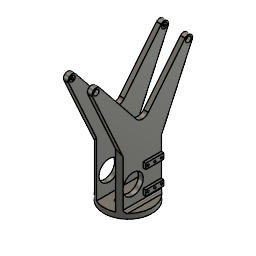
Base plate PiPER v7 V2 (Autodesk Fusion 360 design; units mm, degrees)
part number: 2025-11-21-17-17-18-129
Autodesk Fusion 360 part; units mm, degrees
sketch "Sketch1" plane through (0, 0, 0) normal (0, 1, 0) x (1, 0, 0)
  circle A0 centre (0, 0) radius 28.5
  circle A1 centre (11.6913, -6.75) radius 2
  circle A2 centre (11.6913, 6.75) radius 2
  circle A3 centre (0, 13.5) radius 2
  circle A4 centre (-11.6913, 6.75) radius 2
  circle A5 centre (-11.6913, -6.75) radius 2
  circle A6 centre (0, -13.5) radius 2
  spline S0 degree 5 poles (2.6699, 14.6244) (2.6558, 14.5371) (2.6371, 14.3587) (2.6331, 14.0815) (2.6571, 13.7017) (2.6824, 13.2287) (2.655, 12.7724) (2.5426, 12.3428) (2.3408, 11.943) (2.0817, 11.5691) (1.8161, 11.2121) (1.5972, 10.8601) (1.4651, 10.5006) (1.4272, 10.1227) (1.4558, 9.719) (1.5099, 9.2874) (1.5508, 8.8329) (1.5594, 8.369) (1.5542, 7.9199) (1.5754, 7.5127) (1.6684, 7.1694) (1.868, 6.8996) (2.1791, 6.6899) (2.5766, 6.5084) (3.0214, 6.3189) (3.4712, 6.0933) (3.8935, 5.8234) (4.2785, 5.5351) (4.6335, 5.2747) (4.9749, 5.0918) (5.3217, 5.0256) (5.6878, 5.086) (6.0765, 5.2462) (6.4838, 5.4621) (6.8992, 5.6875) (7.3078, 5.8897) (7.692, 6.069) (8.0346, 6.2519) (8.3242, 6.4724) (8.5585, 6.7591) (8.7505, 7.1166) (8.9281, 7.5201) (9.1243, 7.9319) (9.3686, 8.3127) (9.6795, 8.6342) (10.0543, 8.8943) (10.4711, 9.1133) (10.896, 9.3237) (11.2884, 9.5617) (11.6068, 9.8592) (11.815, 10.2333) (11.8842, 10.6878) (11.7936, 11.2159) (11.5324, 11.8027) (11.1006, 12.4275) (10.5109, 13.0664) (9.7861, 13.6938) (8.957, 14.2835) (8.0599, 14.8102) (7.1342, 15.2509) (6.2204, 15.5861) (5.3571, 15.801) (4.5795, 15.8872) (3.9162, 15.8439) (3.3874, 15.6792) (3.003, 15.4088) (2.8094, 15.1239) (2.7213, 14.8822) (2.6839, 14.7116) (2.6699, 14.6244) knots 0 0 0 0 0 0 0.01538462 0.03076923 0.04615385 0.06153846 0.07692308 0.09230769 0.10769231 0.12307692 0.13846154 0.15384615 0.16923077 0.18461538 0.2 0.21538462 0.23076923 0.24615385 0.26153846 0.27692308 0.29230769 0.30769231 0.32307692 0.33846154 0.35384615 0.36923077 0.38461538 0.4 0.41538462 0.43076923 0.44615385 0.46153846 0.47692308 0.49230769 0.50769231 0.52307692 0.53846154 0.55384615 0.56923077 0.58461538 0.6 0.61538462 0.63076923 0.64615385 0.66153846 0.67692308 0.69230769 0.70769231 0.72307692 0.73846154 0.75384615 0.76923077 0.78461538 0.8 0.81538462 0.83076923 0.84615385 0.86153846 0.87692308 0.89230769 0.90769231 0.92307692 0.93846154 0.95384615 0.96923077 0.98461538 1 1 1 1 1 1
  spline S1 degree 5 poles (-14, -5) (-13.9174, -4.9685) (-13.7535, -4.8955) (-13.5115, -4.7604) (-13.1946, -4.5497) (-12.7976, -4.2913) (-12.3888, -4.0869) (-11.9605, -3.9694) (-11.5134, -3.9443) (-11.06, -3.9818) (-10.618, -4.0333) (-10.2037, -4.0469) (-9.8264, -3.9814) (-9.4801, -3.8253) (-9.1448, -3.5987) (-8.7981, -3.3361) (-8.4249, -3.0734) (-8.0275, -2.834) (-7.6359, -2.614) (-7.2939, -2.392) (-7.0431, -2.1399) (-6.9092, -1.8321) (-6.8831, -1.4578) (-6.9247, -1.0228) (-6.9831, -0.5428) (-7.0126, -0.0405) (-6.99, 0.4602) (-6.9328, 0.9377) (-6.8848, 1.3754) (-6.8971, 1.7624) (-7.0131, 2.096) (-7.2485, 2.3828) (-7.5816, 2.6393) (-7.9722, 2.8841) (-8.3751, 3.1311) (-8.7545, 3.3839) (-9.1019, 3.6269) (-9.4316, 3.8323) (-9.7674, 3.9728) (-10.1328, 4.0323) (-10.5384, 4.0199) (-10.9767, 3.9719) (-11.4313, 3.9359) (-11.8832, 3.9571) (-12.3172, 4.0656) (-12.7299, 4.2601) (-13.1279, 4.5116) (-13.5225, 4.7744) (-13.9249, 4.9951) (-14.3417, 5.1222) (-14.7698, 5.1155) (-15.198, 4.9481) (-15.6101, 4.6056) (-15.9876, 4.086) (-16.3128, 3.3996) (-16.5713, 2.5695) (-16.7522, 1.6281) (-16.8484, 0.6152) (-16.856, -0.4251) (-16.7748, -1.4471) (-16.6081, -2.406) (-16.3626, -3.2611) (-16.0484, -3.9776) (-15.6793, -4.5304) (-15.2723, -4.9061) (-14.8459, -5.1037) (-14.5024, -5.129) (-14.249, -5.0843) (-14.0826, -5.0315) (-14, -5) knots 0 0 0 0 0 0 0.01538462 0.03076923 0.04615385 0.06153846 0.07692308 0.09230769 0.10769231 0.12307692 0.13846154 0.15384615 0.16923077 0.18461538 0.2 0.21538462 0.23076923 0.24615385 0.26153846 0.27692308 0.29230769 0.30769231 0.32307692 0.33846154 0.35384615 0.36923077 0.38461538 0.4 0.41538462 0.43076923 0.44615385 0.46153846 0.47692308 0.49230769 0.50769231 0.52307692 0.53846154 0.55384615 0.56923077 0.58461538 0.6 0.61538462 0.63076923 0.64615385 0.66153846 0.67692308 0.69230769 0.70769231 0.72307692 0.73846154 0.75384615 0.76923077 0.78461538 0.8 0.81538462 0.83076923 0.84615385 0.86153846 0.87692308 0.89230769 0.90769231 0.92307692 0.93846154 0.95384615 0.96923077 0.98461538 1 1 1 1 1 1
  spline S2 degree 5 poles (11.3301, -9.6244) (11.2616, -9.5686) (11.1164, -9.4631) (10.8784, -9.3211) (10.5375, -9.152) (10.1152, -8.9374) (9.7338, -8.6855) (9.4179, -8.3733) (9.1726, -7.9987) (8.9783, -7.5873) (8.8019, -7.1788) (8.6066, -6.8132) (8.3612, -6.5192) (8.0529, -6.2973) (7.689, -6.1203) (7.2882, -5.9514) (6.8741, -5.7595) (6.4681, -5.535) (6.0817, -5.3059) (5.7185, -5.1207) (5.3747, -5.0296) (5.0412, -5.0675) (4.7041, -5.2321) (4.3481, -5.4856) (3.9617, -5.7761) (3.5414, -6.0528) (3.0965, -6.2836) (2.6543, -6.4729) (2.2513, -6.6501) (1.9222, -6.8543) (1.6914, -7.1215) (1.5607, -7.4688) (1.5051, -7.8856) (1.4884, -8.3462) (1.4759, -8.8186) (1.4467, -9.2736) (1.4099, -9.696) (1.397, -10.0842) (1.4432, -10.4452) (1.5743, -10.7914) (1.7879, -11.1365) (2.0486, -11.4921) (2.3071, -11.8678) (2.5147, -12.2697) (2.6377, -12.6998) (2.6756, -13.1545) (2.6568, -13.6249) (2.6265, -14.098) (2.6365, -14.5569) (2.7349, -14.9813) (2.9548, -15.3487) (3.3138, -15.6359) (3.8165, -15.8215) (4.4553, -15.8887) (5.2122, -15.8272) (6.0604, -15.6359) (6.9661, -15.3219) (7.8914, -14.8987) (8.7961, -14.3852) (9.6406, -13.8039) (10.3878, -13.18) (11.0055, -12.5399) (11.4689, -11.9095) (11.7631, -11.3134) (11.8849, -10.7732) (11.8429, -10.305) (11.693, -9.995) (11.5277, -9.7978) (11.3987, -9.6801) (11.3301, -9.6244) knots 0 0 0 0 0 0 0.01538462 0.03076923 0.04615385 0.06153846 0.07692308 0.09230769 0.10769231 0.12307692 0.13846154 0.15384615 0.16923077 0.18461538 0.2 0.21538462 0.23076923 0.24615385 0.26153846 0.27692308 0.29230769 0.30769231 0.32307692 0.33846154 0.35384615 0.36923077 0.38461538 0.4 0.41538462 0.43076923 0.44615385 0.46153846 0.47692308 0.49230769 0.50769231 0.52307692 0.53846154 0.55384615 0.56923077 0.58461538 0.6 0.61538462 0.63076923 0.64615385 0.66153846 0.67692308 0.69230769 0.70769231 0.72307692 0.73846154 0.75384615 0.76923077 0.78461538 0.8 0.81538462 0.83076923 0.84615385 0.86153846 0.87692308 0.89230769 0.90769231 0.92307692 0.93846154 0.95384615 0.96923077 0.98461538 1 1 1 1 1 1
  circle A7 centre (0, 0) radius 13.5 construction
  circle A8 centre (0, -13.5) radius 1.7
  circle A9 centre (0, 13.5) radius 1.7
  line L0 (-7, 0) -> (-16.8414, 0) construction
  circle A10 centre (-11.9207, 0) radius 2.1654
  circle A11 centre (5.9604, -10.3236) radius 2.1654
  circle A12 centre (5.9604, 10.3236) radius 2.1654
  point P0 (2.5359, 12.3923)
  point P1 (1.5359, 10.6603)
  point P2 (1.7679, 7.0622)
  point P3 (5.2321, 5.0622)
  point P4 (8.4641, 6.6603)
  point P5 (9.4641, 8.3923)
  point P6 (11.3301, 9.6244)
  point P7 (11.4641, 11.8564)
  point P8 (4.5359, 15.8564)
  point P9 (3.5, 6.0622)
  point P10 (7.0147, 5.7421)
  point P11 (1.5439, 8.8149)
  point P12 (-12, -4)
  point P13 (-10, -4)
  point P14 (-8.4059, -3.0704)
  point P15 (-7, -2)
  point P16 (-7, 0)
  point P17 (-7, 2)
  point P18 (-8.4801, 3.2039)
  point P19 (-10, 4)
  point P20 (-12, 4)
  point P21 (-14, 5)
  point P22 (-16, 4)
  point P23 (-16, -4)
  point P24 (9.4641, -8.3923)
  point P25 (8.4641, -6.6603)
  point P26 (6.862, -5.7445)
  point P27 (5.2321, -5.0622)
  point P28 (3.5, -6.0622)
  point P29 (1.7679, -7.0622)
  point P30 (1.4654, -8.946)
  point P31 (1.5359, -10.6603)
  point P32 (2.5359, -12.3923)
  point P33 (2.6699, -14.6244)
  point P34 (4.5359, -15.8564)
  point P35 (11.4641, -11.8564)
  dimension "d3" = 57
  dimension "d9" = 4
  dimension "d11" = 360
  dimension "d33" = 27
  dimension "d255" = 3.4
  dimension "d256" = 3.4
  constraint coincident A0.centre A7.centre
  constraint concentric A0 A7
  constraint concentric A6 A8
  constraint concentric A3 A9
  constraint coincident P16 L0.start
  constraint coincident S1 L0.end
  constraint horizontal L0
  constraint midpoint L0 A10.centre
  measures "d3" diameter of A0
  measures "d9" diameter of A1
  measures "d33" diameter of A7
  measures "d255" diameter of A8
  measures "d256" diameter of A9
extrude "Extrude7" add sketch "Sketch1" against normal blind 4 contours S0 | S1 | S2 | A10 | A11 | A12 makes body 1 at (9.8365, -1.0048, 8.738) makes body 2 at (-12.8395, -1.0048, -4.3378) makes body 3 at (2.6491, -1.0048, -12.8883)
scale "Scale1" factor 1 about (-14, -4, 5) bodies 2
scale "Scale2" factor 0.9 about (-11.9207, 0, 0) bodies 2
scale "Scale3" factor 0.9 about (5.9604, 0, 10.3236) bodies 1
scale "Scale4" factor 0.9 about (5.9604, 0, -10.3236) bodies 3
extrude "Extrude35" add sketch "Sketch1" along normal blind 2 separate body contours A3 | A6 makes body 4 at (1.9975, 1.3333, -13.4003) makes body 5 at (1.9975, 1.3333, 13.5997)
extrude "Extrude24" add sketch "Sketch1" along normal blind 6 contours A0 | A1 | A2 | A4 | A5 | S0 | S1 | S2 | A10 | A11 | A12 bodies 1 4 5 2 3
sketch "Sketch13" plane through (0, 6, 0) normal (0, 1, 0) x (-1, 0, 0)
  circle A0 centre (0, -13.5) radius 2
  circle A1 centre (0, 13.5) radius 2
  line L0 (0, 0) -> (9, 0)
  line L1 (14, 0) -> (14, -21.9089)
  line L2 (14, 0) -> (14, 21.9089)
  line L3 (0, 40) -> (0, -40)
  line L4 (-14, 0) -> (-14, 21.9089)
  line L5 (-14, 0) -> (-14, -21.9089)
  line L6 (8.9562, 50) -> (17.0461, 50)
  line L7 (17.0461, 50) -> (17.0461, -50)
  line L8 (17.0461, -50) -> (11.4128, -50)
  line L9 (-8.9562, 50) -> (-17.0461, 50)
  line L10 (-17.0461, 50) -> (-17.0461, -50)
  line L11 (-17.0461, -50) -> (-11.4128, -50)
  circle A2 centre (0, 0) radius 28.5
  line L12 (-11.4128, 50.6271) -> (-11.4128, -50)
  line L13 (11.4128, 50.6271) -> (11.4128, -50)
  line L14 (0, -40) -> (-11.5, -40) construction
  line L15 (-11.5, -40) -> (-17.044, -40)
  dimension "d228" = 5.544
  constraint coincident L0.start A2.centre
  constraint horizontal L0
  constraint perpendicular L0 L1
  constraint parallel L1 L2
  constraint vertical L3
  constraint symmetric L1.start L3 L4.start
  constraint symmetric L1.end L3 L5.end
  constraint symmetric L2.end L3 L4.end
  constraint horizontal L6
  constraint vertical L7
  constraint horizontal L8
  constraint symmetric L3 L6.start L9.start
  constraint symmetric L3 L6.end L9.end
  constraint symmetric L3 L7.end L10.end
  constraint symmetric L3 L8.end L11.end
  constraint perpendicular L11 L12
  constraint symmetric L3 L11.end L8.end
  constraint symmetric L3 L12.start L13.start
  constraint perpendicular L10 L14
  constraint perpendicular L10 L15
  measures "d228" distance of L14.end L15.end
extrude "Extrude25" add sketch "Sketch13" along normal blind 80 contours L10 A2 L12 | L7 A2 L13 bodies 1
sketch "Sketch14" plane through (0, 0, 0) normal (1, 0, 0) x (0, 1, 0)
  circle A0 centre (30, 11) radius 12
  circle A1 centre (43.5, -11.75) radius 1.25
  circle A2 centre (16.5, -11.75) radius 1.25
  circle A3 centre (16.5, -3.75) radius 1.25
  circle A4 centre (43.5, -3.75) radius 1.25
  line L0 (13, -1) -> (47, -1)
  line L1 (40.5, -22.4834) -> (19.5106, -22.4834)
  line L2 (19.5106, -22.4834) -> (19.5106, -1)
  line L3 (19.5106, -1) -> (40.5, -1)
  line L4 (40.5, -1) -> (40.5, -22.4834)
  line L5 (40.5, -22.4834) -> (47, -22.4834)
  line L6 (19.5106, -22.4834) -> (13, -22.4834)
  line L7 (47, -22.4834) -> (47, -1)
  line L8 (13, -22.4834) -> (13, -1)
  circle A5 centre (43.5, -19.75) radius 1.25
  circle A6 centre (16.5, -19.75) radius 1.25
  circle A7 centre (76, 0) radius 2
  circle A8 centre (43.5, -3.75) radius 2.3049
  circle A9 centre (16.5, -19.75) radius 2.3049
  circle A10 centre (43.5, -19.75) radius 2.3049
  circle A11 centre (43.5, -11.75) radius 2.3049
  circle A12 centre (16.5, -11.75) radius 2.3049
  circle A13 centre (16.5, -3.75) radius 2.3049
  dimension "d160" = 24
  dimension "d194" = 4
  constraint horizontal L0
  constraint horizontal L1
  constraint vertical L2
  constraint horizontal L3
  constraint vertical L4
  constraint coincident L0 L2.end
  constraint perpendicular L2 L6
  constraint perpendicular L0 L8
  constraint concentric A4 A8
  measures "d160" diameter of A0
  measures "d194" diameter of A7
extrude "Extrude28" cut sketch "Sketch14" along normal through all and the other way through all contours A0 bodies 1
extrude "Extrude29" add sketch "Sketch14" along normal blind 3.1 from surface at 17.0461 separate body contours L0 L2 L6 L8 | L0 L4 L5 L7 | A8 | A9 | A10 | A11 | A12 | A13 makes body 6 at (17.0461, 46.25, -11.7445) makes body 7 at (17.0461, 13.75, -11.7445)
extrude "Extrude38" cut sketch "Sketch14" along normal blind 37 contours A1 | A2 | A3 | A4 | A5 | A6 bodies 1
extrude "Extrude39" cut sketch "Sketch14" along normal blind 13 contours A8 | A9 | A10 | A11 | A12 | A13 bodies 1
sketch "Sketch15" plane through (0, 0, 0) normal (1, 0, 0) x (0, 1, 0)
  line L0 (86, 0) -> (146, 0)
  circle A0 centre (146, -54.6955) radius 1.35
  circle A1 centre (146, -54.6955) radius 5
  line L1 (86, 0) -> (149.1345, -50.8)
  line L2 (63.7979, -22.8269) -> (143.9312, -59.2474)
  line L3 (86, 0) -> (149.1345, 50.8)
  line L4 (63.7979, 22.8269) -> (143.9312, 59.2474)
  circle A2 centre (146, 54.6955) radius 1.35
  circle A3 centre (146, 54.6955) radius 5
  line L5 (86, 0) -> (63.7979, -22.8269)
  line L6 (86, 0) -> (63.7979, 22.8269)
  line L7 (146, 0) -> (146, -54.6955) construction
  line L8 (63.7979, -22.8269) -> (63.7979, 22.8269)
  line L9 (86, 0) -> (63.7979, 0)
  circle A4 centre (146, -54.6955) radius 3.2713
  circle A5 centre (146, 54.6955) radius 3.2713
  dimension "d181" = 60
  dimension "d183" = 2.7
  dimension "d184" = 10
  dimension "d229" = 54.6955
  dimension "d261" = 2.7
  constraint horizontal L0
  constraint concentric A0 A1
  constraint coincident A1 L1.end
  constraint tangent A1 L1
  constraint coincident A1 L2.end
  constraint tangent A1 L2
  constraint symmetric L0 A0 A2
  constraint symmetric L0 A1 A3
  constraint symmetric L0 L1.end L3.end
  constraint symmetric L0 L2.start L4.start
  constraint symmetric L0 L2.end L4.end
  constraint perpendicular L0 L7
  constraint coincident A0.centre A1.centre
  constraint midpoint L8 L9.end
  constraint symmetric L0 A4 A5
  measures "d181" distance of L0.end L0.start
  measures "d183" diameter of A0
  measures "d184" diameter of A1
  measures "d229" distance of L0.end A0.centre
  measures "d261" diameter of A2
extrude "Extrude31" add sketch "Sketch15" along normal up to surface (5.6333 mm away) from surface at 11.4128 contours A1 | A1 L1 L2 L5 | L3 L4 A3 L6 | A3 bodies 1
extrude "Extrude32" add sketch "Sketch15" along normal up to surface (5.6333 mm away) from surface at -17.0461 contours A1 | A1 L1 L2 L5 | L3 L4 A3 L6 | A3 bodies 1
fillet "Fillet9" radius 9 2 edges at (14.2295, 86, 0) (-14.2295, 86, 0) on bodies 1
combine "Combine3" operation add target body 1 tool bodies 6 7
hole "Hole10" at (17.0461, 165.1165, 54.6955) direction (-1, 0, 0) diameter 2.529 depth 50 tip angle 180 bodies 1
thread "Thread1" "ISO Metric profile 3.0 M3x0.5 M3x0.5 6H" thread offset 0 thread depth 7.4
hole "Hole11" at (17.0461, 146.6665, -54.6955) direction (-1, 0, 0) diameter 2.671 depth 60 tip angle 180 bodies 1
thread "Thread2" "ISO Metric profile 3.0 M3x0.35 M3x0.35 6H" thread offset 0 thread depth 7.4
fillet "Fillet10" radius 3 2 edges at (-17.0461, 6, 0) (17.0461, 6, 0) on bodies 1
extrude "Extrude40" add sketch "Sketch15" along normal blind 1.5 from surface at 11.413 separate body contours A4 | A5 makes body 8 at (11.913, 147.7749, 51.9475) makes body 9 at (11.913, 147.7749, -57.4435)
extrude "Extrude41" add sketch "Sketch15" against normal blind 1.5 from surface at -11.413 contours A4 | A5 bodies 1
combine "Combine4" operation add target body 1 tool bodies 8 9
sketch "Sketch16" plane through (0, 0, 0) normal (1, 0, 0) x (0, 1, 0)
  line L0 (125, 0) -> (-20, 0)
  circle A0 centre (107.6752, 23.6627) radius 3.5
  circle A1 centre (107.6752, -23.6627) radius 3.5
  dimension "d200" = 7
  constraint horizontal L0
  constraint symmetric L0 A0 A1
  measures "d200" diameter of A0
extrude "Extrude34" [suppressed]
hole "Hole8" [suppressed]
hole "Hole9" [suppressed]
equation "bearing_ID = 12 mm"
equation "bearing_OD = 32 mm"
equation "bearing_H = 10 mm"
equation "d229 = ( 109.391 / 2 ) * 1 mm"
equation "d249 = ( 22.826 / 2 ) * 1 mm"
equation "d252 = ( -22.826 / 2 ) * 1 mm"
